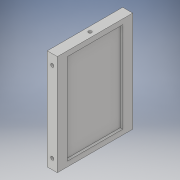
# Autodesk Inventor part: BatteryHighSide
Saved by Autodesk Inventor 2019 (Build 230136000, 136)
## iProperties
Created: 2017-11-10
Part Number: BatteryHighSide
Material: Generic
Document SubType Name: Modeling
Designer: james
Density: 1 g/cm^3
Appearance: Default
Author: james
Autodesk Inventor part; units mm, degrees
ref_plane "YZ Plane" through (0, 0, 0) normal (1, 0, 0) x (0, 1, 0)
ref_plane "XZ Plane" through (0, 0, 0) normal (0, 1, 0) x (-1, 0, 0)
ref_plane "XY Plane" through (0, 0, 0) normal (0, 0, 1) x (1, 0, 0)
sketch "Sketch1" plane through (0, 0, 0) normal (0, 1, 0) x (-1, 0, 0)
  line L0 (7.3766, 22.0919) -> (-5.3234, 22.0919)
  line L1 (-5.3234, 22.0919) -> (-5.3234, -73.1581)
  line L2 (-5.3234, -73.1581) -> (7.3766, -73.1581)
  line L3 (7.3766, -73.1581) -> (7.3766, 22.0919)
  point P0 (0, 0)
  dimension "d0" = 12.7
  dimension "d1" = 95.25
  constraints: 8 end point, 2 parallel, 1 horizontal, 1 perpendicular
  measures "d0" distance of L0.start L0.end
  measures "d1" distance of L0.end L1.end
extrude "Extrusion1" add sketch "Sketch1" along normal blind 127
sketch "Sketch2" plane through (-7.3766, 0, 22.0919) normal (0, 0, 1) x (1, 0, 0)
  line L0 (12.7, 0) -> (12.7, 127) projected
  line L1 (12.7, 127) -> (0, 127) projected
  line L2 (0, 0) -> (12.7, 0) projected
  line L3 (0, 0) -> (0, 127) projected
  point P0 (7.3766, 0)
  point P1 (6.35, 114.3)
  point P2 (6.35, 12.7)
  dimension "d4" = 6.35
  dimension "d5" = 12.7
  dimension "d6" = 12.7
  dimension "d7" = 6.35
  measures "d4" distance from line of L0 point (6.35, 114.3)
  measures "d5" distance from line of L1 point (6.35, 114.3)
  measures "d6" distance from line of L2 point (6.35, 12.7)
  measures "d7" distance from line of L3 point (6.35, 12.7)
hole "Hole1" at (-1.0266, 114.3, 22.0919) at (-1.0266, 12.7, 22.0919) direction (0, 0, -1) diameter 4.0386 depth 12.7 tip angle 118
sketch "Sketch3" plane through (5.3234, 0, -73.1581) normal (0, 0, -1) x (-1, 0, 0)
  line L0 (0, 0) -> (12.7, 0) projected
  line L1 (12.7, 0) -> (12.7, 127) projected
  line L2 (0, 127) -> (12.7, 127) projected
  point P0 (5.3234, 0)
  point P1 (6.35, 114.3)
  point P2 (6.35, 12.7)
  dimension "d15" = 12.7
  dimension "d16" = 6.35
  dimension "d17" = 6.35
  dimension "d18" = 12.7
  measures "d15" distance from line of L0 point (6.35, 12.7)
  measures "d16" distance from line of L1 point (6.35, 12.7)
  measures "d17" distance from line of L1 point (6.35, 114.3)
  measures "d18" distance from line of L2 point (6.35, 114.3)
hole "Hole2" at (-1.0266, 114.3, -73.1581) at (-1.0266, 12.7, -73.1581) direction (0, 0, 1) diameter 4.0386 depth 12.7 tip angle 118
sketch "Sketch4" plane through (5.3234, 0, 22.0919) normal (1, 0, 0) x (0, 0, -1)
  line L0 (12.7, 120.65) -> (82.55, 120.65)
  line L1 (82.55, 120.65) -> (82.55, 6.35)
  line L2 (82.55, 6.35) -> (12.7, 6.35)
  line L3 (12.7, 6.35) -> (12.7, 120.65)
  line L4 (95.25, 127) -> (0, 127) projected
  line L5 (95.25, 0) -> (0, 0) projected
  line L6 (95.25, 0) -> (95.25, 127) projected
  line L7 (0, 0) -> (0, 127) projected
  point P0 (22.0919, 0)
  dimension "d26" = 6.35
  dimension "d27" = 6.35
  dimension "d28" = 12.7
  dimension "d29" = 12.7
  constraints: 8 end point, 2 parallel, 1 horizontal, 1 perpendicular
  measures "d26" distance between parallel lines of L4 L0
  measures "d27" distance between parallel lines of L5 L2
  measures "d28" distance between parallel lines of L6 L1
  measures "d29" distance between parallel lines of L7 L3
extrude "Extrusion2" cut sketch "Sketch4" against normal blind 3.175 contours L0 L1 L2 L3
sketch "Sketch5" plane through (0, 127, 0) normal (0, 1, 0) x (1, 0, 0)
  line L0 (-7.3766, -22.0919) -> (5.3234, -22.0919) projected
  line L1 (5.3234, 73.1581) -> (-7.3766, 73.1581) projected
  line L2 (-7.3766, 73.1581) -> (-7.3766, -22.0919) projected
  point P0 (0, 0)
  point P1 (-1.0266, 25.5331)
  dimension "d32" = 95.25
  dimension "d33" = 6.35
  dimension "d34" = 47.625
  measures "d32" distance between parallel lines of L0 L1
  measures "d33" distance from line of L2 point (-1.027, 25.533)
  measures "d34" distance from line of L0 point (-1.027, 25.533)
hole "Hole3" at (-1.0266, 127, -25.5331) direction (0, -1, 0) diameter 4.0386 depth 25.4 tip angle 118
sketch "Sketch6" plane through (0, 0, 0) normal (0, -1, 0) x (1, 0, 0)
  line L0 (-7.3766, -73.1581) -> (-7.3766, 22.0919) projected
  line L1 (-7.3766, 22.0919) -> (5.3234, 22.0919) projected
  line L2 (5.3234, -73.1581) -> (-7.3766, -73.1581) projected
  point P0 (0, 0)
  point P1 (-1.0266, -3.3081)
  point P2 (-1.0266, -47.7581)
  dimension "d42" = 6.35
  dimension "d43" = 6.35
  dimension "d44" = 25.4
  dimension "d45" = 25.4
  measures "d42" distance from line of L0 point (-1.027, -47.758)
  measures "d43" distance from line of L0 point (-1.027, -3.308)
  measures "d44" distance from line of L1 point (-1.027, -3.308)
  measures "d45" distance from line of L2 point (-1.027, -47.758)
hole "Hole4" at (-1.0266, 0, -3.3081) at (-1.0266, 0, -47.7581) direction (0, 1, 0) diameter 4.0386 depth 12.7 tip angle 118
body "Solid1"
